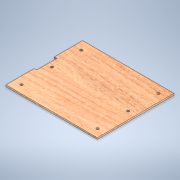
# Autodesk Inventor part: Front plane
Saved by Autodesk Inventor 2020.2 (Build 242310000, 310)
## iProperties
Created: 2020-03-05
Part Number: Front plane
Material: Wood (Birch)
Document SubType Name: Modeling
Designer: sdekr
Density: 0.55 g/cm^3
Appearance: Birch - Natural Polished
Author: sdekr
Autodesk Inventor part; units mm, degrees
ref_plane "YZ Plane" through (0, 0, 0) normal (1, 0, 0) x (0, 1, 0)
ref_plane "XZ Plane" through (0, 0, 0) normal (0, 1, 0) x (-1, 0, 0)
ref_plane "XY Plane" through (0, 0, 0) normal (0, 0, 1) x (1, 0, 0)
sketch "Sketch1" plane through (0, 0, 0) normal (0, 1, 0) x (-1, 0, 0)
  line L0 (-90, 75) -> (90, 75)
  line L1 (90, 75) -> (90, -75)
  line L2 (90, -75) -> (-90, -75)
  line L3 (-90, -75) -> (-90, 75)
  line L4 (-90, 75) -> (90, -75) construction
  line L5 (90, 75) -> (-90, -75) construction
  point P0 (0, 0)
  dimension "d0" = 180
  dimension "d1" = 150
  constraints: 12 end point, 2 midpoint, 2 parallel, 1 horizontal, 1 perpendicular
  measures "d0" distance of L1.end L2.end
  measures "d1" distance of L0.end L1.end
extrude "Extrusion1" add sketch "Sketch1" along normal blind 3
offset faces "Size1" outward 0.5 faces at (-30, 1, 75) (30, 1, -75)
sketch "Sketch2" plane through (0, 0, 0) normal (0, -1, 0) x (1, 0, 0)
  line L0 (-90, -75.5) -> (-90, 75.5) projected
  line L1 (-90, 20) -> (-85, 20)
  line L2 (-85, 20) -> (-85, -20)
  line L3 (-85, -20) -> (-90, -20)
  line L4 (-90, -20) -> (-90, 20)
  point P0 (0, 0)
  point P1 (-90, -77.5)
  point P2 (-90, 77.5)
  point P3 (-85, 0)
  point P4 (-90, 0)
  dimension "d6" = 40
  dimension "d7" = 5
  constraints: 8 end point, 2 midpoint, 2 parallel, 1 horizontal, 1 horizontal alignment, 1 perpendicular, 1 point on line
  measures "d6" distance of L1.end L2.end
  measures "d7" distance of L2.end L3.end
extrude "Extrusion2" cut sketch "Sketch2" against normal blind 10
sketch "Sketch3" plane through (0, 0, 0) normal (0, -1, 0) x (1, 0, 0)
  circle A0 centre (75, 60) radius 2.4 projected
  circle A1 centre (75, 0) radius 2.4 projected
  circle A2 centre (75, -60) radius 2.4 projected
  circle A3 centre (-75, 60) radius 2.4 projected
  circle A4 centre (-75, 0) radius 2.4 projected
  circle A5 centre (-75, -57.6) radius 2.4
  point P0 (0, 0)
  dimension "d10" = 4.8
  constraints: 1 centre point
  measures "d10" diameter of A5
extrude "Extrusion3" cut sketch "Sketch3" against normal blind 10
body "Solid1"
